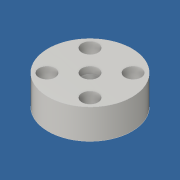
# Autodesk Inventor part: rotBaseMagnetMount
Saved by Autodesk Inventor 2016 (Build 200138000, 138)
## iProperties
Created: 2015-10-04
Part Number: rotBaseMagnetMount
Material: ABS-Kunststoff
Document SubType Name: Modeling
Designer: 4ndreas
Density: 1.06 g/cm^3
Appearance: Glatt - weiß
Mass: 7.94642 g
Surface Area: 31.7458 cm^2
Volume: 7.49663 cm^3
Author: 4ndreas
Autodesk Inventor part; units mm, degrees
ref_plane "YZ Plane" through (0, 0, 0) normal (1, 0, 0) x (0, 1, 0)
ref_plane "XZ Plane" through (0, 0, 0) normal (0, 1, 0) x (-1, 0, 0)
ref_plane "XY Plane" through (0, 0, 0) normal (0, 0, 1) x (1, 0, 0)
sketch "Skizze1" plane through (0, 0, 0) normal (0, 0, 1) x (1, 0, 0)
  circle A0 centre (0, 0) radius 15.5
  dimension "d0" = 31
  constraints: 1 centre point, 1 coincident
  measures "d0" diameter of A0
extrude "Extrusion1" add sketch "Skizze1" along normal blind 11
sketch "Skizze2" plane through (0, 0, 11) normal (0, 0, 1) x (1, 0, 0)
  line L0 (-2.5, -2.5) -> (2.5, -2.5)
  line L1 (2.5, -2.5) -> (2.5, 2.5)
  line L2 (2.5, 2.5) -> (-2.5, 2.5)
  line L3 (-2.5, 2.5) -> (-2.5, -2.5)
  line L4 (-2.5, -2.5) -> (2.5, 2.5) construction
  line L5 (2.5, -2.5) -> (-2.5, 2.5) construction
  circle A0 centre (0, 0) radius 3
  dimension "d3" = 5
  dimension "d14" = 6
  constraints: 12 end point, 2 midpoint, 2 parallel, 2 perpendicular, 1 centre point, 1 coincident, 1 horizontal
  measures "d3" distance between parallel lines of L3 L1
  measures "d14" diameter of A0
extrude "Extrusion2" cut sketch "Skizze2" against normal blind 2.5 contours A0 L3 L2 L1 L0 | L0 A0 | A0 L3 | L1 A0 | A0 L2
sketch "Skizze3" plane through (0, 0, 11) normal (0, 0, 1) x (1, 0, 0)
  circle A0 centre (0, 0) radius 11.25
  line L0 (-7.955, -7.955) -> (7.955, -7.955)
  line L1 (7.955, -7.955) -> (7.955, 7.955)
  line L2 (7.955, 7.955) -> (-7.955, 7.955)
  line L3 (-7.955, 7.955) -> (-7.955, -7.955)
  line L4 (-7.955, -7.955) -> (7.955, 7.955) construction
  line L5 (7.955, -7.955) -> (-7.955, 7.955) construction
  dimension "d6" = 22.5
  constraints: 12 end point, 2 midpoint, 2 parallel, 2 perpendicular, 1 coincident, 1 horizontal, 3 other
hole "Bohrung1" at (-7.955, -7.955, 11) at (7.955, -7.955, 11) at (7.955, 7.955, 11) at (-7.955, 7.955, 11) direction (0, 0, -1) diameter 3 end through all counterbore diameter 6 counterbore depth 5
